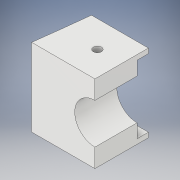
# Autodesk Inventor part: AA016
Saved by Autodesk Inventor 2017 SP1 (Build 210196100, 196)
## iProperties
Created: 2017-09-29
Part Number: AA016
Material: ABS Plastic
Document SubType Name: Modeling
Designer: Zach
Density: 1.06 g/cm^3
Appearance: CR White
Author: Zach
Autodesk Inventor part; units mm, degrees
ref_plane "YZ Plane" through (0, 0, 0) normal (1, 0, 0) x (0, 1, 0)
ref_plane "XZ Plane" through (0, 0, 0) normal (0, 1, 0) x (-1, 0, 0)
ref_plane "XY Plane" through (0, 0, 0) normal (0, 0, 1) x (1, 0, 0)
sketch "Sketch1" plane through (0, 0, 0) normal (0, 0, 1) x (1, 0, 0)
  line L0 (0, 0) -> (70, 0)
  line L1 (70, 0) -> (70, 77.5)
  line L2 (70, 77.5) -> (0, 77.5)
  line L3 (0, 77.5) -> (0, 0)
  dimension "d0" = 70
  dimension "d1" = 77.5
  constraints: 8 end point, 2 parallel, 1 horizontal, 1 perpendicular
  measures "d0" distance of L2.end L1.end
  measures "d1" distance of L1.end L0.end
extrude "Extrusion1" add sketch "Sketch1" along normal blind 95
sketch "Sketch3" plane through (0, 0, 95) normal (0, 0, 1) x (1, 0, 0)
  line L0 (0, 0) -> (70, 0) projected
  line L1 (70, 77.5) -> (0, 77.5) projected
  line L2 (70, 0) -> (35, 0)
  line L3 (35, 0) -> (35, 77.5)
  line L4 (35, 77.5) -> (70, 77.5)
  line L5 (70, 77.5) -> (70, 0)
  constraints: 8 end point, 2 parallel, 1 horizontal, 1 midpoint, 1 perpendicular
extrude "Extrusion3" cut sketch "Sketch3" against normal through all
sketch "Sketch4" plane through (0, 77.5, 95) normal (0, 1, 0) x (1, 0, 0)
  line L0 (0, 95) -> (0, 0) projected
  line L1 (0, 0) -> (-12.5, 0)
  line L2 (35, 95) -> (0, 95) projected
  arc A0 (-12.5, 0) -> (0, 95) centre (-1145.4326, 197.3924) ccw
  line L3 (-12.5, -10) -> (35, -10) construction
  dimension "d9" = 1150
  dimension "d54" = 47.5
  dimension "d55" = 10
  constraints: 4 end point, 2 horizontal, 2 point on circle, 2 vertical alignment, 1 centre point
  measures "d9" radius of A0
  measures "d54" distance of L3.start L3.end
  measures "d55" distance between parallel lines of L1 L3
extrude "Extrusion4" add sketch "Sketch4" against normal blind 77.5
sketch "Sketch5" plane through (35, 0, 95) normal (1, 0, 0) x (0, 0, -1)
  line L0 (0, 77.5) -> (0, 86.25)
  line L1 (0, 0) -> (0, -8.75)
  line L2 (0, 0) -> (0, 77.5) projected
  line L3 (95, 77.5) -> (95, 0) projected
  arc A0 (0, 86.25) -> (95, 77.5) centre (152.8838, 1226.0423) ccw
  arc A1 (95, 0) -> (0, -8.75) centre (152.8838, -1148.5423) ccw
  line L4 (0, 77.5) -> (95, 77.5) projected
  line L5 (95, 0) -> (0, 0) projected
  line L6 (-10, 86.25) -> (-10, -8.75) construction
  point P0 (-10, 38.75)
  point P1 (0, 38.75)
  dimension "d14" = 1150
  dimension "d15" = 1150
  dimension "d52" = 10
  dimension "d53" = 95
  constraints: 6 end point, 4 point on circle, 3 horizontal alignment, 3 vertical, 2 centre point, 2 midpoint
  measures "d14" radius of A0
  measures "d15" radius of A1
  measures "d52" distance between parallel lines of L2 L6
  measures "d53" distance of L6.start L6.end
extrude "Extrusion5" add sketch "Sketch5" against normal blind 55 contours L0 A0 L4 | L5 A1 L1
sketch "Sketch6" plane through (-20, 0, 0) normal (0, 1, 0) x (1, 0, 0)
  line L0 (20, 0) -> (0, 0) projected
  line L1 (0, -95) -> (0, 0) projected
  arc A0 (7.5, -95) -> (20, 0) centre (-1125.4326, 102.3924) ccw projected
  line L2 (7.5, -95) -> (0, -95) projected
extrude "Extrusion6" cut sketch "Sketch6" along normal through all both and the other way through all
fillet "Fillet3" radius 19 2 edges at (-5.299, 80.9203, 47.9253) (-5.299, -3.4203, 47.9253)
sketch "Sketch8" plane through (0, 0, 95) normal (0, 0, 1) x (1, 0, 0)
  line L0 (35, 86.25) -> (35, -8.75) projected
  line L1 (35, 77.5) -> (35, 0) projected
  circle A0 centre (35, 38.75) radius 35
  point P0 (0, 0)
  dimension "d23" = 70
  constraints: 1 centre point, 1 midpoint
  measures "d23" diameter of A0
extrude "Extrusion7" cut sketch "Sketch8" against normal blind 20
sketch "Sketch9" plane through (0, 0, 75) normal (0, 0, 1) x (1, 0, 0)
  line L0 (35, 73.75) -> (35, 3.75) projected
  circle A0 centre (35, 38.75) radius 15.5
  point P0 (0, 0)
  dimension "d26" = 31
  constraints: 1 centre point, 1 midpoint
  measures "d26" diameter of A0
extrude "Extrusion8" cut sketch "Sketch9" against normal blind 20
sketch "Sketch10" plane through (0, 0, 0) normal (0, 0, -1) x (-1, 0, 0)
  line L0 (-35, 77.5) -> (-35, 0) projected
  circle A0 centre (-35, 38.75) radius 12.5
  point P0 (0, 0)
  dimension "d29" = 25
  constraints: 1 centre point, 1 midpoint
  measures "d29" diameter of A0
extrude "Extrusion9" cut sketch "Sketch10" against normal blind 50
sketch "Sketch11" plane through (0, 0, 50) normal (0, 0, -1) x (-1, 0, 0)
  line L0 (-35, 26.25) -> (-35, 51.25) projected
  circle A0 centre (-35, 38.75) radius 2.5
  circle A1 centre (-26.5, 38.75) radius 2
  point P0 (0, 0)
  dimension "d32" = 5
  dimension "d33" = 4
  dimension "d34" = 8.5
  constraints: 3 midpoint, 2 centre point, 2 horizontal alignment
  measures "d32" diameter of A0
  measures "d33" diameter of A1
  measures "d34" distance of A0.centre A1.centre
extrude "Extrusion10" cut sketch "Sketch11" against normal through all
sketch "Sketch12" plane through (0, 0, 55) normal (0, 0, 1) x (1, 0, 0)
  circle A0 centre (26.5, 38.75) radius 2 projected
  circle A1 centre (26.5, 38.75) radius 4.5
  point P0 (0, 0)
  dimension "d37" = 9
  constraints: 1 centre point, 1 coincident
  measures "d37" diameter of A1
extrude "Extrusion11" cut sketch "Sketch12" against normal blind 3
sketch "Sketch14" plane through (0, 0, 50) normal (0, 0, -1) x (-1, 0, 0)
  arc A0 (-35, 36.25) -> (-35, 41.25) centre (-35, 38.75) ccw projected
  circle A1 centre (-35, 38.75) radius 4
  point P0 (0, 0)
  dimension "d40" = 8
  constraints: 1 centre point, 1 coincident
  measures "d40" diameter of A1
extrude "Extrusion12" cut sketch "Sketch14" against normal blind 3
sketch "Sketch15" plane through (0, 0, 75) normal (0, 0, 1) x (1, 0, 0)
  arc A0 (35, 41.25) -> (35, 36.25) centre (35, 38.75) ccw projected
  circle A1 centre (10, 38.75) radius 2.5
  circle A2 centre (22.5, 17.0994) radius 2.5
  circle A3 centre (47.5, 17.0994) radius 2.5
  circle A4 centre (60, 38.75) radius 2.5
  circle A5 centre (47.5, 60.4006) radius 2.5
  circle A6 centre (22.5, 60.4006) radius 2.5
  point P0 (0, 0)
  dimension "d43" = 5
  dimension "d44" = 25
  dimension "d47" = 360
  constraints: 6 centre point, 1 horizontal alignment, 13 other
  measures "d43" diameter of A1
  measures "d44" distance of A0.centre A1.centre
extrude "Extrusion13" cut sketch "Sketch15" against normal blind 25
sketch "Sketch17" plane through (35, 73.75, 95) normal (1, 0, 0) x (0, 0, -1)
  line L0 (90, -60) -> (55, -60)
  line L1 (55, -60) -> (55, -10)
  line L2 (55, -10) -> (90, -10)
  line L3 (90, -10) -> (90, -60)
  line L4 (95, -22.5) -> (95, -47.5) projected
  line L5 (0, 12.5) -> (95, 12.5)
  line L6 (95, 12.5) -> (95, -82.5)
  line L7 (95, -82.5) -> (0, -82.5)
  line L8 (0, -82.5) -> (0, 12.5)
  point P0 (95, -73.75)
  point P1 (90, -35)
  point P2 (95, -35)
  dimension "d62" = 35
  dimension "d63" = 50
  dimension "d64" = 5
  constraints: 16 end point, 4 parallel, 2 horizontal, 2 midpoint, 2 perpendicular, 1 coincident, 1 horizontal alignment, 1 point on line
  measures "d62" distance of L1.end L2.end
  measures "d63" distance of L0.end L1.end
  measures "d64" distance from line of L3 point (95, -73.75)
extrude "Extrusion16" cut sketch "Sketch17" against normal through all
sketch "Sketch18" plane through (35, 13.75, 5) normal (1, 0, 0) x (0, 0, -1)
  line L0 (0, 4) -> (-8, 4)
  line L1 (-8, 4) -> (-8, 46)
  line L2 (-8, 46) -> (0, 46)
  line L3 (0, 46) -> (0, 4)
  line L4 (-35, 37.5) -> (-35, 12.5) projected
  line L5 (0, 12.5) -> (0, 37.5) projected
  point P0 (5, -13.75)
  point P1 (0, 25)
  dimension "d69" = 42
  dimension "d70" = 8
  constraints: 8 end point, 2 midpoint, 2 parallel, 1 horizontal, 1 perpendicular
  measures "d69" distance of L0.end L1.end
  measures "d70" distance of L1.end L2.end
extrude "Extrusion17" cut sketch "Sketch18" against normal blind 25
sketch "Sketch19" plane through (35, 13.75, 5) normal (0, -1, 0) x (1, 0, 0)
  circle A0 centre (-15, 17.5) radius 2.5
  line L0 (0, 35) -> (0, 0) projected
  point P0 (-35, -5)
  point P1 (0, 17.5)
  dimension "d73" = 5
  dimension "d74" = 15
  constraints: 1 centre point, 1 horizontal alignment, 1 midpoint
  measures "d73" diameter of A0
  measures "d74" distance from line of L0 A0.centre
extrude "Extrusion18" cut sketch "Sketch19" against normal through all
sketch "Sketch20" plane through (35, 51.25, 40) normal (1, 0, 0) x (0, 0, -1)
  line L0 (35, -37.5) -> (35, -33.5) projected
  line L1 (0, 12.5) -> (35, 12.5)
  line L2 (35, 12.5) -> (35, -37.5)
  line L3 (35, -37.5) -> (0, -37.5)
  line L4 (0, -37.5) -> (0, 12.5)
  line L5 (34, 11.5) -> (1, 11.5)
  line L6 (1, 11.5) -> (1, -36.5)
  line L7 (1, -36.5) -> (34, -36.5)
  line L8 (34, -36.5) -> (34, 11.5)
  point P0 (40, -51.25)
  dimension "d77" = 1
  constraints: 16 end point, 4 parallel, 2 perpendicular, 1 horizontal, 3 other
  measures "d77" distance between parallel lines of L1 L5
extrude "Extrusion19" cut sketch "Sketch20" against normal through all
body "Solid1"
